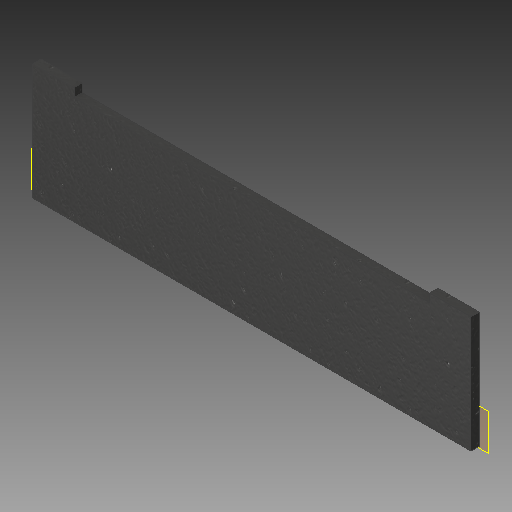
# Autodesk Inventor part: sides
Saved by Autodesk Inventor 2018 (Build 220112000, 112)
## iProperties
Created: 2017-10-09
Part Number: sides
Material: Generic
Document SubType Name: Modeling
Designer: HP
Density: 1 g/cm^3
Appearance: Fine Textured - Black
Author: HP
Autodesk Inventor part; units mm, degrees
ref_plane "YZ Plane" through (0, 0, 0) normal (1, 0, 0) x (0, 1, 0)
ref_plane "XZ Plane" through (0, 0, 0) normal (0, 1, 0) x (-1, 0, 0)
ref_plane "XY Plane" through (0, 0, 0) normal (0, 0, 1) x (1, 0, 0)
ref_plane "Work Plane1" through (0, 0, 0.5) normal (0, 0, 1) x (1, 0, 0)
sketch "Sketch1" plane through (0, 0, 0.5) normal (0, 0, 1) x (1, 0, 0)
  line L0 (250, 0) -> (0, 0) construction
  line L1 (250, 0) -> (250, 20) construction
  line L2 (0, 20) -> (250, 20) construction
  line L3 (0, 0) -> (0, 20) construction
  line L4 (245, 20) -> (153.1686, 20) construction
  line L5 (245, 20) -> (245, 80) construction
  line L6 (153.1686, 80) -> (245, 80) construction
  line L7 (153.1686, 20) -> (153.1686, 80) construction
  line L8 (-7, 0) -> (257, 0)
  line L9 (257, 0) -> (257, 70)
  line L10 (257, 70) -> (232.1, 70)
  line L11 (232.1, 70) -> (232.1, 64.9)
  line L12 (232.1, 64.9) -> (17.9, 64.9)
  line L13 (17.9, 64.9) -> (17.9, 70)
  line L14 (17.9, 70) -> (-7, 70)
  line L15 (-7, 70) -> (-7, 0)
  dimension "d0" = 10
  dimension "d1" = 5.1
  dimension "d2" = 7
  dimension "d3" = 7
  dimension "d4" = 24.9
  dimension "d5" = 24.9
  constraints: 16 end point, 5 perpendicular, 3 point on line, 1 collinear, 1 vertical
  measures "d0" distance between parallel lines of L10 L6
  measures "d1" distance between parallel lines of L12 L10
  measures "d2" distance between parallel lines of L15 L3
  measures "d3" distance between parallel lines of L9 L1
  measures "d4" distance between parallel lines of L13 L15
  measures "d5" distance between parallel lines of L11 L9
extrude "Extrusion1" add sketch "Sketch1" along normal blind 5
equation "\"d1\" = ABS_tolerance + plate_thickness"
equation "\"d5\" = d4"
equation "\"d6\" = plate_thickness"
equation "\"plate_thickness\" = 5"
equation "\"ABS_tolerance\" = 0.1"
equation "\"laser_cutter_thickness\" = 0.1"
equation "\"basic_plate_offser\" = 0.5"
equation "\"basic_plate_offset\" = 0.5"
body "Solid1"
